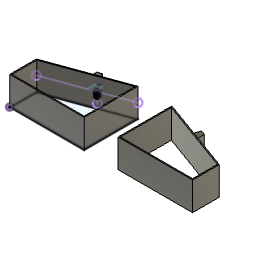
Microfreak Parametric v11 (Autodesk Fusion 360 design; units mm, degrees)
Autodesk Fusion 360 part; units mm, degrees
sketch "Sketch1" plane through (0, 0, 0) normal (0, 0, 1) x (1, 0, 0)
  line L0 (0, 0) -> (131.557, 0)
  line L1 (131.557, 0) -> (131.557, 95)
  line L2 (131.557, 95) -> (0, 47.1172)
  line L3 (0, 0) -> (0, 47.1172)
  line L4 (2, 2) -> (2, 45.7168)
  line L5 (129.557, 92.1437) -> (2, 45.7168)
  line L6 (129.557, 2) -> (129.557, 92.1437)
  line L7 (2, 2) -> (129.557, 2)
  dimension "d12" = 95
  dimension "d13" = 70
  dimension "d15" = 140
  constraint coincident L0.start L3.start
  constraint horizontal L0
  constraint perpendicular L0 L1
  constraint perpendicular L0 L3
  measures "d12" distance of L0.end L1.end
  measures "d13" angle of L1 L2
  measures "d15" distance of L1.end L2.end
extrude "Extrude1" add sketch "Sketch1" along normal blind 50 makes body 1
ref_plane "WorkPlane1" through (65.7785, 47.5, 25) normal (0, 0, -1) x (-1, 0, 0)
sketch "Sketch2" plane through (65.7785, 47.5, 25) normal (0, 0, -1) x (1, 0, 0)
  line L0 (0.1419, -23.6102) -> (13.2976, -28.3985)
  line L1 (65.7785, -47.5) -> (-65.7785, 0.3828)
  line L2 (13.2976, -28.3985) -> (8.1673, -42.4939)
  line L3 (8.1673, -42.4939) -> (0.6497, -39.7577)
  line L4 (0.6497, -39.7577) -> (0.1419, -23.6102)
  dimension "d19" = 14
  dimension "d20" = 15
  dimension "d21" = 8
  constraint collinear L0 L1
  constraint perpendicular L1 L2
  constraint perpendicular L2 L3
  measures "d19" distance of L0.start L0.end
  measures "d20" distance of L0.end L2.end
  measures "d21" distance of L2.end L3.end
extrude "Extrude2" add sketch "Sketch2" along normal blind 17 from surface at 1 bodies 1
mirror "Mirror1" about plane through (65.7785, 47.5, 25) normal (0, 0, -1) of "Extrude2"
ref_plane "WorkPlane3" through (65.7785, 71.0586, 25) normal (-0.34202, 0.939693, 0) x (-0.939693, -0.34202, 0)
sketch "Sketch4" plane through (65.7785, 71.0586, 25) normal (-0.34202, 0.939693, 0) x (-0.939693, -0.34202, 0)
  circle A0 centre (-14.151, -6) radius 3
  line L0 (-14.151, -1) -> (-14.151, -18)
  line L1 (-14.151, -1) -> (-14.151, -6)
  dimension "d31" = 6
  dimension "d34" = 5
  constraint coincident L0.start L1.start
  constraint coincident L0 A0.centre
  constraint coincident A0.centre L1.end
  measures "d31" diameter of A0
  measures "d34" distance of L0.start A0.centre
extrude "Extrude4" cut sketch "Sketch4" along normal blind 15 bodies 1
extrude "Extrude3" cut sketch "Sketch4" along normal blind 15 bodies 1
ref_plane "WorkPlane4" through (161.557, 47.5, 25) normal (1, 0, 0) x (0, 1, 0)
mirror "Mirror2" about plane through (161.557, 47.5, 25) normal (1, 0, 0) of bodies 1 makes body 2
equation "tabHeight = 15 mm" comment "Should not edit this parameter"
equation "tabTopLength = 8 mm" comment "Should not edit this parameter"
equation "tabBottomLength = 14 mm" comment "Should not edit this parameter"
equation "tabSpacer = 2 mm" comment "Should not edit this parameter"
equation "tabCircleRadius = 3 mm" comment "Should not edit this parameter"
equation "tabCircleSpacer = 5 mm" comment "Should not edit this parameter"
equation "tilt = 20 deg" comment "Device tilt"
equation "baseWidth = 50 mm" comment "Stand width"
equation "baseHeight = 95 mm" comment "Stand height"
equation "thickness = 2 mm" comment "Stand thickness"
equation "roundness = 1 mm" comment "Stand roundness"
equation "d12 = baseHeight"
equation "d13 = 90 deg - tilt"
equation "baseLength = 140 mm" comment "Stand length"
equation "d15 = baseLength"
equation "d16 = -thickness"
equation "d17 = baseWidth"
equation "d19 = tabBottomLength"
equation "d20 = tabHeight"
equation "d21 = tabTopLength"
equation "tabWidth = 17 mm" comment "Should not edit this parameter"
equation "d23 = tabSpacer / 2"
equation "d24 = tabWidth"
equation "d31 = tabCircleRadius * 2"
equation "d32 = tabHeight"
equation "d34 = tabCircleSpacer"
equation "d35 = tabHeight"
equation "d37 = tabHeight * 2"
